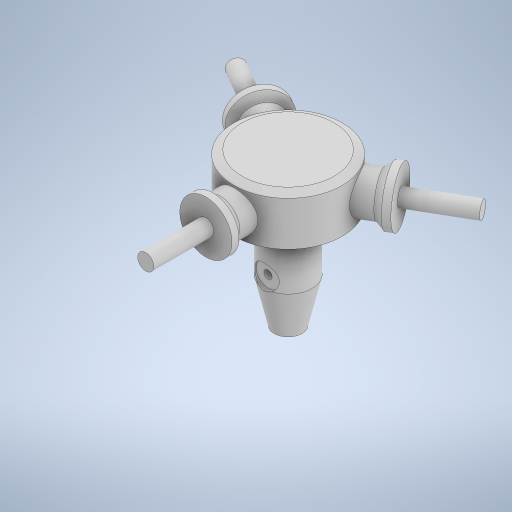
# Autodesk Inventor part: RotorKopf_Hub
Saved by Autodesk Inventor 2023.2 (Build 272271000, 271)
## iProperties
Created: 2023-03-30
Part Number: RotorKopf_Hub
Material: Generisch
Document SubType Name: Modeling
Designer: tadeu
Density: 1 g/cm^3
Appearance: Vorgabe
Author: tadeu
Autodesk Inventor part; units mm, degrees
ref_plane "YZ Plane" through (0, 0, 0) normal (1, 0, 0) x (0, 1, 0)
ref_plane "XZ Plane" through (0, 0, 0) normal (0, 1, 0) x (-1, 0, 0)
sketch "Skizze1" plane through (0, 0, 0) normal (0, 1, 0) x (-1, 0, 0)
  circle A0 centre (0, 0) radius 13.5
  dimension "d0" = 27
  constraints: 1 centre point, 1 coincident
  measures "d0" diameter of A0
extrude "Extrusion1" add sketch "Skizze1" along normal blind 13
chamfer "Fase5" distance 1 distance2 2 1 edges at (13.5, 0, 0) measured on face at (13.5, 0.5, 0)
chamfer "Fase1" distance 2 distance2 1 1 edges at (13.5, 13, 0) measured on face at (13, 13, 0)
sketch "Skizze2" plane through (0, 0, 0) normal (0, -1, 0) x (1, 0, 0)
  circle A0 centre (0, 0) radius 6
  dimension "d6" = 12
  constraints: 1 centre point, 1 coincident
  measures "d6" diameter of A0
extrude "Extrusion2" add sketch "Skizze2" along normal blind 25
chamfer "Fase2" distance 3 angle 45 1 edges at (-6, 0, 0)
chamfer "Fase3" distance 2.5 distance2 11 1 edges at (-6, -25, 0) measured on face at (-5.5, -25, 0)
sketch "Skizze3" plane through (0, -25, 0) normal (0, -1, 0) x (1, 0, 0)
  circle A0 centre (0, 0) radius 3
  dimension "d15" = 6
  constraints: 1 centre point, 1 coincident
  measures "d15" diameter of A0
extrude "Extrusion3" cut sketch "Skizze3" against normal blind 33
sketch "Skizze4" plane through (0, 0, 0) normal (0, 0, 1) x (1, 0, 0)
  circle A0 centre (0, -11.5) radius 1
  line L0 (12.5, 0) -> (-12.5, 0) projected
  line L1 (0, 24.2271) -> (0, -45.182) construction
  circle A1 centre (0, -11.5) radius 3
  point P0 (0, 0)
  dimension "d18" = 2
  dimension "d19" = 11.5
  dimension "d22" = 6
  constraints: 2 centre point, 2 end point, 1 coincident, 1 vertical
  measures "d18" diameter of A0
  measures "d19" distance from line of L0 A0.centre
  measures "d22" diameter of A1
extrude "Extrusion4" cut sketch "Skizze4" along normal through all both and the other way through all contours A0
ref_plane "Arbeitsebene1" through (0, 0, 6) normal (0, 0, 1) x (1, 0, 0)
sketch "Skizze5" plane through (0, 0, 6) normal (0, 0, 1) x (1, 0, 0)
  circle A0 centre (0, -11.5) radius 3
  line L0 (12.5, 0) -> (-12.5, 0) projected
  point P0 (0, 0)
  dimension "d24" = 6
  dimension "d27" = 11.5
  constraints: 1 centre point
  measures "d24" diameter of A0
  measures "d27" distance from line of L0 A0.centre
extrude "Extrusion5" cut sketch "Skizze5" against normal blind 1
mirror "Spiegeln1" about plane through (0, 0, 0) normal (0, 0, 1) of "Extrusion5"
sketch "Skizze6" plane through (0, 0, 0) normal (0, 0, 1) x (1, 0, 0)
  circle A0 centre (0, 6.5) radius 5
  line L0 (-11.5, 13) -> (11.5, 13) projected
  point P0 (0, 0)
  dimension "d28" = 10
  dimension "d44" = 6.5
  constraints: 1 centre point
  measures "d28" diameter of A0
  measures "d44" distance from line of L0 A0.centre
ref_plane "Arbeitsebene2" through (0, 0, 17) normal (0, 0, 1) x (1, 0, 0)
extrude "Extrusion6" add sketch "Skizze6" against normal up to surface from surface at 17 round surface about axis through (0, 0, 0) along (0, 1, 0) radius 13.5 far side no
sketch "Skizze7" plane through (0, 6.5, 17) normal (0, 0, 1) x (1, 0, 0)
  circle A0 centre (0, 0) radius 6.5
  point P0 (0, -6.5)
  dimension "d35" = 13
  constraints: 1 centre point
  measures "d35" diameter of A0
extrude "Extrusion7" add sketch "Skizze7" along normal blind 3.5
chamfer "Fase4" distance 1.75 distance2 1.5 1 edges at (-6.5, 6.5, 17) measured on face at (-6.5, 6.5, 17.5)
sketch "Skizze8" plane through (0, 6.5, 20.5) normal (0, 0, 1) x (1, 0, 0)
  circle A0 centre (0, 0) radius 2
  point P0 (0, -6.5)
  dimension "d45" = 4
  constraints: 1 centre point
  measures "d45" diameter of A0
extrude "Extrusion8" add sketch "Skizze8" along normal blind 15
pattern_circular "Runde Anordnung1" count 3 over 360 about axis through (0, 0, 0) along (0, 1, 0) of "Extrusion7", "Fase4", "Extrusion6", "Extrusion8"
